Autodesk Fusion 360 part; units mm, degrees
(part 3 of 3)
component "Hinge_Pin_D3_R" placed x (1, 0, 0) y (0, 1, 0) z (0, 0, 1) at (0, 0, 0) in component "03_Hinged_Wedgelets"
component "Eclip_DIN6799_2.3_R" placed x (1, 0, 0) y (0, 1, 0) z (0, 0, 1) at (0, 0, 0) in component "03_Hinged_Wedgelets"
component "01_Printed_Chassis_TPU" placed x (1, 0, 0) y (0, 1, 0) z (0, 0, 1) at (0, 0, 0) in component "Wedgelet_L"
component "Tub_TPU" placed x (1, 0, 0) y (0, 1, 0) z (0, 0, 1) at (0, 0, 0) in component "Eclip_DIN6799_2.3_L"
component "Skirt_Plate_1mm_L" placed x (1, 0, 0) y (0, 1, 0) z (0, 0, 1) at (0, 0, 0) in component "03b_Hinged_Skirts"
component "Skirt_Wire_D1.5_L" placed x (1, 0, 0) y (0, 1, 0) z (0, 0, 1) at (0, 0, 0) in component "03b_Hinged_Skirts"
component "Skirt_Clip_PETG_L1" placed x (1, 0, 0) y (0, 1, 0) z (0, 0, 1) at (0, 0, 0) in component "03b_Hinged_Skirts"
component "Skirt_Clip_PETG_L2" placed x (1, 0, 0) y (0, 1, 0) z (0, 0, 1) at (0, 0, 0) in component "03b_Hinged_Skirts"
component "Skirt_Clip_PETG_L3" placed x (1, 0, 0) y (0, 1, 0) z (0, 0, 1) at (0, 0, 0) in component "03b_Hinged_Skirts"
component "Skirt_Clip_PETG_L4" placed x (1, 0, 0) y (0, 1, 0) z (0, 0, 1) at (0, 0, 0) in component "03b_Hinged_Skirts"
component "Skirt_Plate_1mm_R" placed x (1, 0, 0) y (0, 1, 0) z (0, 0, 1) at (0, 0, 0) in component "03b_Hinged_Skirts"
component "Skirt_Wire_D1.5_R" placed x (1, 0, 0) y (0, 1, 0) z (0, 0, 1) at (0, 0, 0) in component "03b_Hinged_Skirts"
component "Skirt_Clip_PETG_R1" placed x (1, 0, 0) y (0, 1, 0) z (0, 0, 1) at (0, 0, 0) in component "03b_Hinged_Skirts"
component "Skirt_Clip_PETG_R2" placed x (1, 0, 0) y (0, 1, 0) z (0, 0, 1) at (0, 0, 0) in component "03b_Hinged_Skirts"
component "Skirt_Clip_PETG_R3" placed x (1, 0, 0) y (0, 1, 0) z (0, 0, 1) at (0, 0, 0) in component "03b_Hinged_Skirts"
component "Skirt_Clip_PETG_R4" placed x (1, 0, 0) y (0, 1, 0) z (0, 0, 1) at (0, 0, 0) in component "03b_Hinged_Skirts"
component "Skirt_Plate_1mm_Rear" placed x (1, 0, 0) y (0, 1, 0) z (0, 0, 1) at (0, 0, 0) in component "03b_Hinged_Skirts"
component "Skirt_Wire_D1.5_Rear" placed x (1, 0, 0) y (0, 1, 0) z (0, 0, 1) at (0, 0, 0) in component "03b_Hinged_Skirts"
component "Skirt_Clip_PETG_Rear1" placed x (1, 0, 0) y (0, 1, 0) z (0, 0, 1) at (0, 0, 0) in component "03b_Hinged_Skirts"
component "Skirt_Clip_PETG_Rear2" placed x (1, 0, 0) y (0, 1, 0) z (0, 0, 1) at (0, 0, 0) in component "03b_Hinged_Skirts"
component "Skirt_Clip_PETG_Rear3" placed x (1, 0, 0) y (0, 1, 0) z (0, 0, 1) at (0, 0, 0) in component "03b_Hinged_Skirts"
component "JGA25_370_400rpm_Front_L" placed x (1, 0, 0) y (0, 1, 0) z (0, 0, 1) at (0, 0, 0) in component "04_Drive_4WD"
component "Wheel_Hub_PETG_Front_L" placed x (1, 0, 0) y (0, 1, 0) z (0, 0, 1) at (0, 0, 0) in component "04_Drive_4WD"
component "Wheel_Tyre_TPU_Front_L" placed x (1, 0, 0) y (0, 1, 0) z (0, 0, 1) at (0, 0, 0) in component "04_Drive_4WD"
component "JGA25_370_400rpm_Front_R" placed x (1, 0, 0) y (0, 1, 0) z (0, 0, 1) at (0, 0, 0) in component "04_Drive_4WD"
component "Wheel_Hub_PETG_Front_R" placed x (1, 0, 0) y (0, 1, 0) z (0, 0, 1) at (0, 0, 0) in component "04_Drive_4WD"
component "Wheel_Tyre_TPU_Front_R" placed x (1, 0, 0) y (0, 1, 0) z (0, 0, 1) at (0, 0, 0) in component "04_Drive_4WD"
component "JGA25_370_400rpm_Rear_L" placed x (1, 0, 0) y (0, 1, 0) z (0, 0, 1) at (0, 0, 0) in component "04_Drive_4WD"
component "Wheel_Hub_PETG_Rear_L" placed x (1, 0, 0) y (0, 1, 0) z (0, 0, 1) at (0, 0, 0) in component "04_Drive_4WD"
component "Wheel_Tyre_TPU_Rear_L" placed x (1, 0, 0) y (0, 1, 0) z (0, 0, 1) at (0, 0, 0) in component "04_Drive_4WD"
component "JGA25_370_400rpm_Rear_R" placed x (1, 0, 0) y (0, 1, 0) z (0, 0, 1) at (0, 0, 0) in component "04_Drive_4WD"
component "Wheel_Hub_PETG_Rear_R" placed x (1, 0, 0) y (0, 1, 0) z (0, 0, 1) at (0, 0, 0) in component "04_Drive_4WD"
component "Wheel_Tyre_TPU_Rear_R" placed x (1, 0, 0) y (0, 1, 0) z (0, 0, 1) at (0, 0, 0) in component "04_Drive_4WD"
component "3S_850mAh_LiPo_ENVELOPE_75x35x25" placed x (1, 0, 0) y (0, 1, 0) z (0, 0, 1) at (0, 0, 0) in component "05_Electronics_ENVELOPES"
component "Skywalker_40A_ESC_55x25x12" placed x (1, 0, 0) y (0, 1, 0) z (0, 0, 1) at (0, 0, 0) in component "05_Electronics_ENVELOPES"
component "ESP32_DevKit_51.5x28.3" placed x (1, 0, 0) y (0, 1, 0) z (0, 0, 1) at (0, 0, 0) in component "05_Electronics_ENVELOPES"
component "DRV8871_L" placed x (1, 0, 0) y (0, 1, 0) z (0, 0, 1) at (0, 0, 0) in component "05_Electronics_ENVELOPES"
component "DRV8871_R" placed x (1, 0, 0) y (0, 1, 0) z (0, 0, 1) at (0, 0, 0) in component "05_Electronics_ENVELOPES"
component "IMU_Foam_Pad_1mm" placed x (1, 0, 0) y (0, 1, 0) z (0, 0, 1) at (0, 0, 0) in component "05_Electronics_ENVELOPES"
component "IMU_GY521_MPU6050_21x16" placed x (1, 0, 0) y (0, 1, 0) z (0, 0, 1) at (0, 0, 0) in component "05_Electronics_ENVELOPES"
component "Hall_Post_PETG" placed x (1, 0, 0) y (0, 1, 0) z (0, 0, 1) at (0, 0, 0) in component "05_Electronics_ENVELOPES"
component "Hall_A3144_TO92" placed x (1, 0, 0) y (0, 1, 0) z (0, 0, 1) at (0, 0, 0) in component "05_Electronics_ENVELOPES"
component "Power_Switch_Link" placed x (1, 0, 0) y (0, 1, 0) z (0, 0, 1) at (0, 0, 0) in component "05_Electronics_ENVELOPES"
named bodies: "Tub_TPU", "Lid_TPU_2mm", "Upright_6061_6mm_L", "Upright_6061_6mm_R", "Weapon_Top_Brace_3mm", "Weapon_Bottom_Brace_3mm", "Beater_Disc_L", "Beater_Disc_R", "Beater_Hub_6061_D30", "Bearing_608_L", "Bearing_608_R", "Spacer_Outer_L_ID8.2_OD11", "Spacer_Inner_ID8.2_OD11", "Spacer_Outer_R_ID8.2_OD11", "Dead_Shaft_M8_12.9", "D3536_1250kV_Can_ENVELOPE", "Motor_Pulley_D26_Groove", "Weapon_Motor_Mount_3mm", "Belt_Upper_ENVELOPE", "Belt_Lower_ENVELOPE", "Wedgelet_L", "Wedgelet_R", "Wedgelet_Block_PETG_L", "Wedgelet_Carrier_PETG_L1", "Wedgelet_Carrier_PETG_L2", "Hinge_Pin_D3_L", "Eclip_DIN6799_2.3_L", "Wedgelet_Block_PETG_R", "Wedgelet_Carrier_PETG_R1", "Wedgelet_Carrier_PETG_R2", "Hinge_Pin_D3_R", "Eclip_DIN6799_2.3_R", "Skirt_Plate_1mm_L", "Skirt_Wire_D1.5_L", "Skirt_Clip_PETG_L1", "Skirt_Clip_PETG_L2", "Skirt_Clip_PETG_L3", "Skirt_Clip_PETG_L4", "Skirt_Plate_1mm_R", "Skirt_Wire_D1.5_R", "Skirt_Clip_PETG_R1", "Skirt_Clip_PETG_R2", "Skirt_Clip_PETG_R3", "Skirt_Clip_PETG_R4", "Skirt_Plate_1mm_Rear", "Skirt_Wire_D1.5_Rear", "Skirt_Clip_PETG_Rear1", "Skirt_Clip_PETG_Rear2", "Skirt_Clip_PETG_Rear3", "JGA25_370_400rpm_Front_L", "Wheel_Hub_PETG_Front_L", "Wheel_Tyre_TPU_Front_L", "JGA25_370_400rpm_Front_R", "Wheel_Hub_PETG_Front_R", "Wheel_Tyre_TPU_Front_R", "JGA25_370_400rpm_Rear_L", "Wheel_Hub_PETG_Rear_L", "Wheel_Tyre_TPU_Rear_L", "JGA25_370_400rpm_Rear_R", "Wheel_Hub_PETG_Rear_R", "Wheel_Tyre_TPU_Rear_R", "3S_850mAh_LiPo_ENVELOPE_75x35x25", "Skywalker_40A_ESC_55x25x12", "ESP32_DevKit_51.5x28.3", "DRV8871_L", "DRV8871_R", "IMU_Foam_Pad_1mm", "IMU_GY521_MPU6050_21x16", "Hall_Post_PETG", "Hall_A3144_TO92", "Power_Switch_Link"
